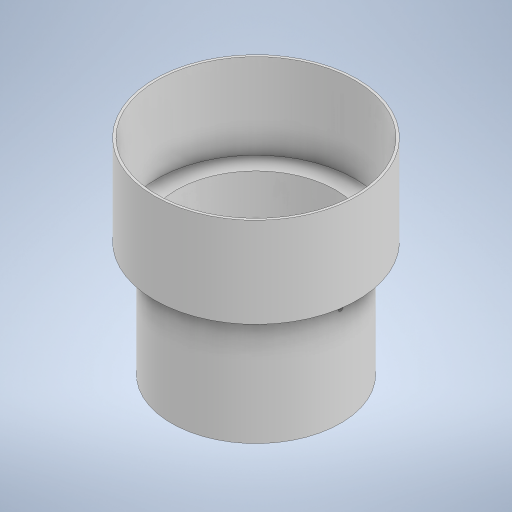
# Autodesk Inventor part: BottomTubeDown
Saved by Autodesk Inventor 2023.2 (Build 272271030, 271C)
## iProperties
Created: 2023-02-12
Part Number: BottomTubeDown
Material: Generic
Document SubType Name: Modeling
Designer: Lukas
Density: 1 g/cm^3
Appearance: Default
polomer: 33.200 mm
drazka: 50.000 mm
pcb: 66.000 mm
tvc_vyska: 17.000 mm
vyska_motor: 34.500 mm
tloustka: 2.000 mm
vyska: 200.000 mm
Author: Lukas
Autodesk Inventor part; units mm, degrees
ref_plane "YZ Plane" through (0, 0, 0) normal (1, 0, 0) x (0, 1, 0)
ref_plane "XZ Plane" through (0, 0, 0) normal (0, 1, 0) x (-1, 0, 0)
ref_plane "XY Plane" through (0, 0, 0) normal (0, 0, 1) x (1, 0, 0)
sketch "Sketch1" plane through (0, 0, 0) normal (1, 0, 0) x (0, 1, 0)
  line L0 (-116.2182, 0) -> (19.3697, 0) projected
  line L1 (-46.9485, -33.2) -> (-46.9485, -41.2)
  line L2 (-11.4485, -41.2) -> (-46.9485, -41.2)
  line L3 (-48.3, -33.2) -> (-60.6, -33.2)
  line L4 (-11.4485, -42.2) -> (-48.9485, -42.2)
  line L5 (-48.9485, -42.2) -> (-48.9485, -35.2)
  line L6 (-48.9485, -35.2) -> (-96.8485, -35.2)
  line L7 (-96.8485, -35.2) -> (-96.8485, -33.2)
  line L8 (-46.9485, -33.2) -> (-48.3, -33.2)
  line L9 (-63.9485, -33.2) -> (-63.9485, -30.2)
  line L10 (-63.9485, -30.2) -> (-65.9485, -30.2)
  line L11 (-65.9485, -30.2) -> (-65.9485, -33.2)
  line L12 (-96.8485, -33.2) -> (-65.9485, -33.2)
  line L13 (-63.9485, -33.2) -> (-60.6, -33.2)
  line L14 (-11.4485, -41.2) -> (-11.4485, -42.2)
  point P0 (0, 0)
  point P1 (-46.9485, -41.7)
  point P2 (-96.8485, -34.2)
  point P3 (-48.9485, -38.7)
  point P4 (-11.4485, -41.7)
  dimension "d43" = 41.2
  dimension "d53" = 33.2
  dimension "d58" = 1
  dimension "d61" = 2
  dimension "d65" = 2
  dimension "d66" = 17
  dimension "d68" = 49.9
  dimension "d69" = 35.5
  dimension "d72" = 2
  dimension "d74" = 42.2
  dimension "d78" = 35.5
  dimension "d79" = 3
  constraints: 28 end point, 5 perpendicular, 3 midpoint, 3 point on line, 2 horizontal, 2 vertical
  measures "d43" distance from line of L2 point (0, 0)
  measures "d53" distance between parallel lines of L0 L3
  measures "d58" distance between parallel lines of L4 L2
  measures "d61" distance between parallel lines of L5 L1
  measures "d65" distance of L9.end L10.end
  measures "d66" distance between parallel lines of L9 L1
  measures "d68" distance between parallel lines of L7 L1
  measures "d69" distance from line of L1 L2.start
  measures "d72" distance between parallel lines of L6 L12
  measures "d74" distance between parallel lines of L0 L4
  measures "d78" distance of point (-46.949, -41.7) point (-11.449, -41.7)
  measures "d79" distance between parallel lines of L13 L10
revolve "Revolution1" add sketch "Sketch1" angle 360 about axis through (0, -10, 0) along (0, 1, 0)
sketch "Sketch2" plane through (0, 0, 0) normal (1, 0, 0) x (0, 1, 0)
  line L0 (-96.8485, -35.2) -> (-96.8485, 35.2) projected
  line L1 (-114.1482, 0) -> (19.0247, 0) projected
  point P0 (0, 0)
  point P1 (-55.4485, 0)
  dimension "d64" = 41.4
  constraints: 1 point on line
  measures "d64" distance from line of L0 point (-55.449, 0)
hole "Hole1" at (0, -55.4485, 0) direction (1, 0, 0) diameter 1.9 depth 40
hole "Hole2" at (0, -55.4485, 0) direction (-1, 0, 0) diameter 1.9 depth 40
fillet "Fillet1" [suppressed]
fillet "Fillet3" radius 3 1 edges at (0, -65.9485, 33.2)
equation "\"gap\" = 0.1"
body "Solid1"
